problem selecting circles_v5 (Autodesk Fusion 360 design; units mm, degrees)
Autodesk Fusion 360 part; units mm, degrees
sketch "stock" plane through (0, 0, 0) normal (0, 0, 1) x (1, 0, 0)
  line L0 (20.1004, -90.6543) -> (-390.4011, -90.6543)
  line L1 (-390.4011, -90.6543) -> (-390.4011, 615.3)
  line L2 (-390.4011, 615.3) -> (0.0808, 615.3)
  line L3 (0.0808, 615.3) -> (20.1004, -90.6543)
  constraint horizontal L2
  constraint vertical L1
  constraint horizontal L0
extrude "stock body extrude Feature" add sketch "stock" along normal blind 3.175
sketch "test for circle drill multiselect op" plane through (0, 0, 0) normal (0, 0, 1) x (1, 0, 0) in component "b top component"
  circle A0 centre (-79.3194, 2.4644) radius 1.005
  circle A1 centre (-70.6806, 2.4644) radius 1.005
  circle A2 centre (-59.3194, 2.4644) radius 1.005
  circle A3 centre (-50.6806, 2.4644) radius 1.005
  circle A4 centre (-39.3194, 2.4644) radius 1.005
  circle A5 centre (-30.6806, 2.4644) radius 1.005
  circle A6 centre (-19.3194, 2.4644) radius 1.005
  circle A7 centre (-10.6806, 2.4644) radius 1.005
  circle A8 centre (-2.4644, 15.6806) radius 1.005
  circle A9 centre (-2.4644, 24.3194) radius 1.005
  circle A10 centre (-2.4644, 35.6806) radius 1.005
  circle A11 centre (-2.4644, 44.3194) radius 1.005
  circle A12 centre (-79.3194, 57.5356) radius 1.005
  circle A13 centre (-70.6806, 57.5356) radius 1.005
  circle A14 centre (-59.3194, 57.5356) radius 1.005
  circle A15 centre (-50.6806, 57.5356) radius 1.005
  circle A16 centre (-39.3194, 57.5356) radius 1.005
  circle A17 centre (-30.6806, 57.5356) radius 1.005
  circle A18 centre (-19.3194, 57.5356) radius 1.005
  circle A19 centre (-10.6806, 57.5356) radius 1.005
  circle A20 centre (-87.5356, 15.6806) radius 1.005
  circle A21 centre (-87.5356, 24.3194) radius 1.005
  circle A22 centre (-87.5356, 35.6806) radius 1.005
  circle A23 centre (-87.5356, 44.3194) radius 1.005
sketch "test for rectangle contour multiselect op" plane through (0, 0, 0) normal (0, 0, 1) x (1, 0, 0)
  line L0 (-51, 32) -> (-17, 32)
  line L1 (-17, 32) -> (-17, -2)
  line L2 (-17, -2) -> (-51, -2)
  line L3 (-51, -2) -> (-51, 32)
  line L4 (-79, 22) -> (-72, 22)
  line L5 (-72, 22) -> (-72, 16)
  line L6 (-72, 16) -> (-79, 16)
  line L7 (-79, 16) -> (-79, 22)
  line L8 (-60, 46) -> (-53, 46)
  line L9 (-53, 46) -> (-53, 36)
  line L10 (-53, 36) -> (-60, 36)
  line L11 (-60, 36) -> (-60, 46)
  dimension "d138" = 7
  dimension "d139" = 7
  constraint horizontal L0
  constraint vertical L1
  constraint horizontal L2
  constraint vertical L3
  constraint horizontal L4
  constraint vertical L5
  constraint horizontal L6
  constraint vertical L7
  constraint horizontal L8
  constraint vertical L9
  constraint horizontal L10
  constraint vertical L11
  measures "d138" distance of L4.start L4.end
  measures "d139" distance of L8.start L8.end
component "b top component" placed x (1, 0, 0) y (0, 1, 0) z (0, 0, 1) at (0, 0, 0)
equation "b_ = 5 mm" comment "added by script"
named bodies: "stock"
